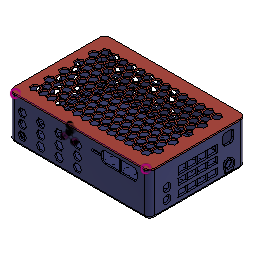
M5xxx (Autodesk Fusion 360 design; units mm, degrees)
Autodesk Fusion 360 part; units mm, degrees
note: some values were not read from the file. Set by a fixed rule: which face or edge a step refers to.
(part 1 of 4)
sketch "Sketch2" plane through (0, 0, 0) normal (0, 0, 1) x (1, 0, 0) in component "PCB-M5000"
  line L0 (110, -75) -> (-110, -75)
  line L1 (-110, -75) -> (-110, 75)
  line L2 (-110, 75) -> (110, 75)
  line L3 (110, 75) -> (110, -75)
  line L4 (110, -75) -> (-110, 75) construction
  line L5 (-110, -75) -> (110, 75) construction
  circle A0 centre (-105, 70) radius 1.75
  circle A1 centre (105, 70) radius 1.75
  circle A2 centre (105, -70) radius 1.75
  circle A3 centre (15, -70) radius 1.75
  circle A4 centre (-105, -70) radius 1.75
  line L6 (0, 0) -> (0, 75) construction
  line L7 (0, 0) -> (-110, 0) construction
  line L8 (125, 32) -> (100, 32)
  line L9 (100, 32) -> (100, -32)
  line L10 (100, -32) -> (125, -32)
  line L11 (125, -32) -> (125, 32)
  line L12 (125, 32) -> (100, -32) construction
  line L13 (100, 32) -> (125, -32) construction
  line L14 (110, -56) -> (97, -56)
  line L15 (97, -56) -> (97, -44)
  line L16 (97, -44) -> (110, -44)
  line L17 (110, -44) -> (110, -56)
  line L18 (110, -56) -> (97, -44) construction
  line L19 (97, -56) -> (110, -44) construction
  line L20 (-110, -62.5) -> (-103, -62.5)
  line L21 (-103, -62.5) -> (-103, -57.5)
  line L22 (-103, -57.5) -> (-110, -57.5)
  line L23 (-110, -57.5) -> (-110, -62.5)
  line L24 (-110, -62.5) -> (-103, -57.5) construction
  line L25 (-103, -62.5) -> (-110, -57.5) construction
  point P0 (112.5, 0)
  point P1 (103.5, -50)
  point P2 (-106.5, -60)
  dimension "d1" = 220
  dimension "d2" = 150
  dimension "d3" = 5
  dimension "d4" = 5
  dimension "d5" = 3.5
  dimension "d6" = 90
  dimension "d10" = 64
  dimension "d11" = 25
  dimension "d13" = 10
  dimension "d18" = 12
  dimension "d19" = 13
  dimension "d20" = 25
  dimension "d26" = 7
  dimension "d27" = 15
  dimension "d28" = 5
  constraint perpendicular L0 L1
  constraint parallel L0 L2
  constraint parallel L1 L3
  constraint horizontal L0
  constraint coincident L4 L6.start
  constraint coincident L5 L6.start
  constraint coincident L6.start L7.start
  constraint equal A3 A4
  constraint equal A2 A3
  constraint equal A1 A2
  constraint equal A0 A1
  constraint midpoint L2 L6.end
  constraint midpoint L1 L7.end
  constraint symmetric A0.centre A1.centre L6
  constraint symmetric A0.centre A4.centre L7
  constraint symmetric A2.centre A4.centre L6
  constraint horizontal A2.centre A3.centre
  constraint perpendicular L8 L9
  constraint parallel L8 L10
  constraint parallel L9 L11
  constraint horizontal L8
  constraint coincident L12 P0
  constraint coincident L13 P0
  constraint horizontal L6.start P0
  constraint perpendicular L14 L15
  constraint parallel L14 L16
  constraint parallel L15 L17
  constraint horizontal L14
  constraint coincident L3 L14.start
  constraint coincident L18 P1
  constraint coincident L19 P1
  constraint perpendicular L20 L21
  constraint parallel L20 L22
  constraint parallel L21 L23
  constraint horizontal L20
  constraint coincident L1 L20.start
  constraint coincident L24 P2
  constraint coincident L25 P2
  measures "d1" distance of L1.end L2.end
  measures "d2" distance of L0.end L1.end
  measures "d3" distance of L1 A0.centre
  measures "d4" distance of L2 A0.centre
  measures "d5" diameter of A0
  measures "d6" distance of A2.centre A3.centre
  measures "d10" distance of L8.end L9.end
  measures "d11" distance of L9.end L10.end
  measures "d13" distance of L3 L9
  measures "d18" distance of L14.end L15.end
  measures "d19" distance of L14.start L14.end
  measures "d20" distance of L0 P1
  measures "d26" distance of L21.end L22.end
  measures "d27" distance of L0 P2
  measures "d28" distance of L20.end L21.end
extrude "Extrude1" add sketch "Sketch2" against normal blind 1.6 contours L0 L1 L2 L3 L8 L9 L10 L14 L15 L16 L20 L21 L22 | L3 L14 L15 L16 L17 | L1 L20 L21 L22 L23 | L3 L8 L9 L10 makes body 1 in component "PCB-M5000"
extrude "Extrude2" add sketch "Sketch2" along normal blind 10.4 contours L3 L8 L9 L10 | L3 L8 L10 L11 bodies 1 in component "PCB-M5000"
fillet "Fillet1" radius 5 4 edges at (110, -75, -0.8) (-110, -75, -0.8) (-110, 75, -0.8) (110, 75, -0.8) on bodies 1 in component "PCB-M5000"
extrude "Extrude4" add sketch "Sketch2" along normal blind 11 contours L3 L14 L15 L16 L17 bodies 1 in component "PCB-M5000"
sketch "Sketch3" plane through (110, 0, 0) normal (1, 0, 0) x (0, 1, 0) in component "PCB-M5000"
  line L0 (-32, 0) -> (-44, 0)
  line L1 (-44, 0) -> (-44, 11)
  line L2 (-44, 11) -> (-56, 11)
  line L3 (-56, 11) -> (-56, 0)
  line L4 (-56, 0) -> (-70, 0)
  line L5 (-70, 0) -> (-70, -1.6)
  line L6 (-70, -1.6) -> (70, -1.6)
  circle A0 centre (-50, 6.5) radius 4.5
  line L7 (-50, 6.5) -> (-50, 11) construction
  line L8 (70, -1.6) -> (70, 0)
  line L9 (70, 0) -> (32, 0)
  line L10 (32, 0) -> (-32, 0)
  dimension "d23" = 9
  constraint tangent L2 A0
  constraint coincident A0.centre L7.start
  constraint midpoint L2 L7.end
  constraint vertical L7
  measures "d23" diameter of A0
extrude "Extrude5" add sketch "Sketch3" along normal blind 10 contours A0 bodies 1 in component "PCB-M5000"
extrude "Extrude6" add sketch "Sketch2" along normal blind 7.5 contours L1 L20 L21 L22 L23 bodies 1 in component "PCB-M5000"
sketch "Sketch4" plane through (-110, 0, 0) normal (-1, 0, 0) x (0, -1, 0) in component "PCB-M5000"
  line L0 (-70, 0) -> (-70, -1.6)
  line L1 (-70, -1.6) -> (70, -1.6)
  line L2 (70, -1.6) -> (70, 0)
  line L3 (70, 0) -> (62.5, 0)
  line L4 (62.5, 0) -> (62.5, 7.5)
  line L5 (62.5, 7.5) -> (57.5, 7.5)
  line L6 (57.5, 7.5) -> (57.5, 0)
  line L7 (57.5, 0) -> (-70, 0)
  circle A0 centre (60, 7.5) radius 1.75
  point P0 (60, 0)
  dimension "d31" = 3.5
  dimension "d243" = 7.5
  constraint vertical A0.centre P0
  measures "d31" diameter of A0
  measures "d243" distance of A0.centre P0
extrude "Extrude7" add sketch "Sketch4" along normal blind 10 contours L5 A0 | L5 A0 bodies 1 in component "PCB-M5000"
ref_plane "WorkPlane1" through (0, 0, 31.6) normal (0, 0, 1) x (1, 0, 0) in component "M2000"
sketch "Sketch1" plane through (0, 0, 31.6) normal (0, 0, 1) x (1, 0, 0) in component "M2000"
  line L0 (110, -75) -> (10, -75)
  line L1 (10, -75) -> (10, 75)
  line L2 (10, 75) -> (110, 75)
  line L3 (110, 75) -> (110, -75)
  line L4 (110, -75) -> (10, 75) construction
  line L5 (10, -75) -> (110, 75) construction
  line L6 (-105, 75) -> (105, 75)
  line L7 (105, -75) -> (-105, -75)
  line L8 (110, 70) -> (110, 32)
  circle A0 centre (105, -70) radius 1.75
  circle A1 centre (15, -70) radius 1.75
  circle A2 centre (105, 70) radius 1.75
  line L9 (125, -32) -> (125, 32)
  line L10 (125, 32) -> (100, 32)
  line L11 (100, 32) -> (100, -32)
  line L12 (100, -32) -> (125, -32)
  line L13 (95, -75) -> (35, -75)
  line L14 (35, -75) -> (35, -55)
  line L15 (35, -55) -> (95, -55)
  line L16 (95, -55) -> (95, -75)
  line L17 (95, -75) -> (35, -55) construction
  line L18 (35, -75) -> (95, -55) construction
  line L19 (110, 40) -> (90, 40)
  line L20 (90, 40) -> (90, 60)
  line L21 (90, 60) -> (110, 60)
  line L22 (110, 60) -> (110, 40)
  line L23 (110, 40) -> (90, 60) construction
  line L24 (90, 40) -> (110, 60) construction
  line L25 (34.5, -75) -> (19.5, -75)
  line L26 (19.5, -75) -> (19.5, -70)
  line L27 (19.5, -70) -> (34.5, -70)
  line L28 (34.5, -70) -> (34.5, -75)
  line L29 (34.5, -75) -> (19.5, -70) construction
  line L30 (19.5, -75) -> (34.5, -70) construction
  circle A3 centre (15, -60) radius 1.6
  point P0 (60, 0)
  point P1 (65, -65)
  point P2 (100, 50)
  point P3 (27, -72.5)
  dimension "d35" = 100
  dimension "d40" = 60
  dimension "d52" = 20
  dimension "d53" = 20
  dimension "d54" = 25
  dimension "d60" = 5
  dimension "d62" = 3.2
  dimension "d63" = 5
  dimension "d64" = 15
  dimension "d67" = 55
  dimension "d68" = 20
  dimension "d69" = 15
  dimension "d70" = 17
  constraint perpendicular L0 L1
  constraint parallel L0 L2
  constraint parallel L1 L3
  constraint horizontal L0
  constraint coincident L4 P0
  constraint coincident L5 P0
  constraint collinear L2 L6
  constraint collinear L0 L7
  constraint collinear L3 L8
  constraint perpendicular L13 L14
  constraint parallel L13 L15
  constraint parallel L14 L16
  constraint horizontal L13
  constraint coincident L17 P1
  constraint coincident L18 P1
  constraint midpoint L17 P1
  constraint coincident L0 L13.start
  constraint perpendicular L19 L20
  constraint parallel L19 L21
  constraint parallel L20 L22
  constraint horizontal L19
  constraint coincident L8 L19.start
  constraint coincident L23 P2
  constraint coincident L24 P2
  constraint perpendicular L25 L26
  constraint parallel L25 L27
  constraint parallel L26 L28
  constraint horizontal L25
  constraint coincident L29 P3
  constraint coincident L30 P3
  constraint coincident L27.end L28.start
  constraint coincident L7 L13.end
  constraint coincident L13.end L14.start
  constraint coincident L0 L25.end
  measures "d35" distance of L1.end L2.end
  measures "d40" distance of L14.end L15.end
  measures "d52" distance of L19.end L20.end
  measures "d53" distance of L19.start L19.end
  measures "d54" distance of L2 P2
  measures "d60" distance of L25.end L26.end
  measures "d62" diameter of A3
  measures "d63" distance of L1 A3.centre
  measures "d64" distance of L0 A3.centre
  measures "d67" distance of L1 P1
  measures "d68" distance of L14.end L13.end
  measures "d69" distance of L25.start L25.end
  measures "d70" horizontal distance of L0.end P3
extrude "Extrude1'" add sketch "Sketch1" along normal blind 1.6 separate body contours L0 L1 L2 L3 L6 L7 L8 L10 L11 L12 L14 L15 L16 L19 L20 L21 L26 L27 L28 | L3 L10 L11 L12 | L0 L7 L13 L14 L15 L16 | L3 L8 L19 L20 L21 L22 | L0 L7 L25 L26 L27 L28 | A3 makes body 2 in component "M2000"
extrude "Extrude2'" add sketch "Sketch1" along normal blind 12 contours L3 L10 L11 L12 | L3 L9 L10 L12 bodies 2 in component "M2000"
extrude "Extrude3" add sketch "Sketch1" along normal blind 20 from surface at 1.6 contours L0 L7 L13 L14 L15 L16 | L3 L8 L19 L20 L21 L22 bodies 2 in component "M2000"
extrude "Extrude6'" add sketch "Sketch1" along normal blind 35 contours A3 bodies 2 in component "M2000"
sketch "Sketch2 (2)" plane through (0, -75, 0) normal (0, -1, 0) x (1, 0, 0) in component "M2000"
  line L0 (10, 31.6) -> (110, 31.6)
  line L1 (110, 33.2) -> (95, 33.2)
  line L2 (95, 33.2) -> (95, 53.2)
  line L3 (95, 53.2) -> (35, 53.2)
  line L4 (35, 53.2) -> (35, 33.2)
  line L5 (35, 33.2) -> (10, 33.2)
  line L6 (10, 33.2) -> (10, 31.6)
  line L7 (93.8, 53.2) -> (36.2, 53.2)
  line L8 (36.2, 53.2) -> (36.2, 34.2)
  line L9 (36.2, 34.2) -> (93.8, 34.2)
  line L10 (93.8, 34.2) -> (93.8, 53.2)
  line L11 (93.8, 53.2) -> (36.2, 34.2) construction
  line L12 (36.2, 53.2) -> (93.8, 34.2) construction
  line L13 (110, 31.6) -> (110, 33.2)
  point P0 (65, 43.7)
  dimension "d46" = 1.2
  dimension "d47" = 1.2
  dimension "d48" = 19
  constraint perpendicular L7 L8
  constraint parallel L7 L9
  constraint parallel L8 L10
  constraint horizontal L7
  constraint coincident L3 L7.start
  constraint coincident L11 P0
  constraint coincident L12 P0
  measures "d46" distance of L2 L10
  measures "d47" distance of L4 L8
  measures "d48" distance of L7 L9
extrude "Extrude4'" add sketch "Sketch2 (2)" along normal blind 10 contours L3 L7 L8 L9 L10 bodies 2 in component "M2000"
sketch "Sketch3 (2)" plane through (110, 0, 0) normal (1, 0, 0) x (0, 1, 0) in component "M2000"
  line L0 (32, 31.6) -> (75, 31.6)
  line L1 (75, 31.6) -> (75, 33.2)
  line L2 (75, 33.2) -> (60, 33.2)
  line L3 (60, 33.2) -> (60, 53.2)
  line L4 (60, 53.2) -> (40, 53.2)
  line L5 (40, 53.2) -> (40, 33.2)
  line L6 (40, 33.2) -> (32, 33.2)
  line L7 (32, 33.2) -> (32, 31.6)
  line L8 (59, 53.2) -> (41, 53.2)
  line L9 (41, 53.2) -> (41, 34.2)
  line L10 (41, 34.2) -> (59, 34.2)
  line L11 (59, 34.2) -> (59, 53.2)
  line L12 (59, 53.2) -> (41, 34.2) construction
  line L13 (41, 53.2) -> (59, 34.2) construction
  point P0 (50, 43.7)
  dimension "d55" = 19
  dimension "d56" = 1
  dimension "d57" = 1
  constraint perpendicular L8 L9
  constraint parallel L8 L10
  constraint parallel L9 L11
  constraint horizontal L8
  constraint coincident L4 L8.start
  constraint coincident L12 P0
  constraint coincident L13 P0
  measures "d55" distance of L8.start L10.end
  measures "d56" distance of L3 L11
  measures "d57" distance of L5 L9
extrude "Extrude5'" add sketch "Sketch3 (2)" along normal blind 10 contours L4 L8 L9 L10 L11 bodies 2 in component "M2000"
fillet "Fillet1'" radius 5 8 edges at (36.2, -80, 53.2) (36.2, -80, 34.2) (93.8, -80, 34.2) (93.8, -80, 53.2) (115, 41, 53.2) (115, 59, 53.2) (115, 59, 34.2) (115, 41, 34.2) on bodies 2 in component "M2000"
fillet "Fillet2" radius 5 4 edges at (10, -75, 32.4) (10, 75, 32.4) (110, 75, 32.4) (110, -75, 32.4) on bodies 2 in component "M2000"
extrude "Extrude7'" add sketch "Sketch1" along normal blind 12.6 from surface at 1.6 contours L0 L7 L25 L26 L27 L28 bodies 2 in component "M2000"
sketch "Sketch4 (2)" plane through (0, -75, 0) normal (0, -1, 0) x (1, 0, 0) in component "M2000"
  line L0 (19.5, 33.2) -> (15, 33.2)
  line L1 (15, 33.2) -> (15, 31.6)
  line L2 (15, 31.6) -> (105, 31.6)
  line L3 (105, 33.2) -> (95, 33.2)
  line L4 (95, 33.2) -> (95, 53.2)
  line L5 (95, 53.2) -> (88.8, 53.2)
  arc A0 (93.8, 48.2) -> (88.8, 53.2) centre (88.8, 48.2) ccw
  line L6 (93.8, 48.2) -> (93.8, 39.2)
  arc A1 (88.8, 34.2) -> (93.8, 39.2) centre (88.8, 39.2) ccw
  line L7 (88.8, 34.2) -> (41.2, 34.2)
  arc A2 (36.2, 39.2) -> (41.2, 34.2) centre (41.2, 39.2) ccw
  line L8 (36.2, 39.2) -> (36.2, 48.2)
  arc A3 (41.2, 53.2) -> (36.2, 48.2) centre (41.2, 48.2) ccw
  line L9 (41.2, 53.2) -> (35, 53.2)
  line L10 (35, 53.2) -> (35, 33.2)
  line L11 (35, 33.2) -> (34.5, 33.2)
  line L12 (34.5, 33.2) -> (34.5, 45.8)
  line L13 (34.5, 45.8) -> (19.5, 45.8)
  line L14 (19.5, 45.8) -> (19.5, 33.2)
  line L15 (21.4, 42) -> (32.6, 42)
  arc A4 (32.6, 42) -> (32.6, 45.8) centre (32.6, 43.9) ccw
  line L16 (32.6, 45.8) -> (21.4, 45.8)
  arc A5 (21.4, 45.8) -> (21.4, 42) centre (21.4, 43.9) ccw
  line L17 (21.4, 43.9) -> (32.6, 43.9) construction
  line L18 (27, 43.9) -> (27, 31.6) construction
  line L19 (105, 31.6) -> (105, 33.2)
  point P0 (27, 31.6)
  dimension "d76" = 3.8
  constraint tangent L15 A4
  constraint tangent A4 L16
  constraint parallel L15 L16
  constraint tangent L16 A5
  constraint tangent L15 A5
  constraint parallel L0 L17
  constraint midpoint L17 L18.start
  constraint coincident P0 L18.end
  constraint vertical L18
  constraint coincident L13 L16.end
  constraint tangent L12 A4
  measures "d76" diameter of A4
extrude "Extrude8" add sketch "Sketch4 (2)" along normal blind 10 contours L13 L15 A4 L16 A5 bodies 2 in component "M2000"
ref_plane "WorkPlane1" through (0, 0, -7.6) normal (0, 0, -1) x (-1, 0, 0) in component "M5xxx-base"
sketch "Sketch1 (2)" plane through (7.5, 0, -7.6) normal (0, 0, -1) x (1, 0, 0) in component "M5xxx-base"
  line L0 (97.5, 75) -> (-112.5, 75)
  arc A0 (102.5, 70) -> (97.5, 75) centre (97.5, 70) ccw
  arc A1 (-112.5, 75) -> (-117.5, 70) centre (-112.5, 70) ccw
  arc A2 (-117.5, -70) -> (-112.5, -75) centre (-112.5, -70) ccw
  line L1 (-112.5, -75) -> (97.5, -75)
  circle A3 centre (-112.5, -70) radius 1.75 construction
  circle A4 centre (97.5, -70) radius 1.75 construction
  arc A5 (97.5, -75) -> (102.5, -70) centre (97.5, -70) ccw
  circle A6 centre (-112.5, 70) radius 1.75 construction
  circle A7 centre (7.5, 70) radius 1.75 construction
  circle A8 centre (97.5, 70) radius 1.75 construction
  line L2 (102.5, 70) -> (102.5, -70)
  line L3 (103.5, 70) -> (103.5, -70)
  arc A9 (97.5, -76) -> (103.5, -70) centre (97.5, -70) ccw
  line L4 (-112.5, -76) -> (97.5, -76)
  arc A10 (-118.5, -70) -> (-112.5, -76) centre (-112.5, -70) ccw
  line L5 (-118.5, 60) -> (-118.5, -70)
  line L6 (-118.5, 70) -> (-118.5, 60)
  arc A11 (-112.5, 76) -> (-118.5, 70) centre (-112.5, 70) ccw
  line L7 (97.5, 76) -> (-112.5, 76)
  arc A12 (103.5, 70) -> (97.5, 76) centre (97.5, 70) ccw
  arc A13 (97.5, -78.4) -> (105.9, -70) centre (97.5, -70) ccw
  line L8 (105.9, 70) -> (105.9, -70)
  arc A14 (105.9, 70) -> (97.5, 78.4) centre (97.5, 70) ccw
  line L9 (97.5, 78.4) -> (-112.5, 78.4)
  arc A15 (-112.5, 78.4) -> (-120.9, 70) centre (-112.5, 70) ccw
  line L10 (-120.9, 70) -> (-120.9, 60)
  line L11 (-120.9, 60) -> (-120.9, -70)
  arc A16 (-120.9, -70) -> (-112.5, -78.4) centre (-112.5, -70) ccw
  line L12 (-112.5, -78.4) -> (97.5, -78.4)
  arc A17 (97.5, -72) -> (99.5, -70) centre (97.5, -70) ccw
  line L13 (99.5, 70) -> (99.5, -70)
  arc A18 (99.5, 70) -> (97.5, 72) centre (97.5, 70) ccw
  line L14 (97.5, 72) -> (-112.5, 72)
  arc A19 (-112.5, 72) -> (-114.5, 70) centre (-112.5, 70) ccw
  line L15 (-114.5, 70) -> (-114.5, 60)
  line L16 (-114.5, 60) -> (-114.5, -70)
  arc A20 (-114.5, -70) -> (-112.5, -72) centre (-112.5, -70) ccw
  line L17 (-112.5, -72) -> (97.5, -72)
  circle A21 centre (97.5, -70) radius 5
  circle A22 centre (97.5, 70) radius 5
  circle A23 centre (-112.5, 70) radius 5
  circle A24 centre (-112.5, -70) radius 5
  circle A25 centre (7.5, 70) radius 5
  line L18 (96.75, -68.701) -> (96, -70)
  line L19 (96, -70) -> (96.75, -71.299)
  line L20 (96.75, -71.299) -> (98.25, -71.299)
  line L21 (98.25, -71.299) -> (99, -70)
  line L22 (99, -70) -> (98.25, -68.701)
  line L23 (98.25, -68.701) -> (96.75, -68.701)
  line L24 (96, 70) -> (96.75, 68.701)
  line L25 (96.75, 68.701) -> (98.25, 68.701)
  line L26 (98.25, 68.701) -> (99, 70)
  line L27 (99, 70) -> (98.25, 71.299)
  line L28 (98.25, 71.299) -> (96.75, 71.299)
  line L29 (96.75, 71.299) -> (96, 70)
  line L30 (8.25, 71.299) -> (6.75, 71.299)
  line L31 (6.75, 71.299) -> (6, 70)
  line L32 (6, 70) -> (6.75, 68.701)
  line L33 (6.75, 68.701) -> (8.25, 68.701)
  line L34 (8.25, 68.701) -> (9, 70)
  line L35 (9, 70) -> (8.25, 71.299)
  line L36 (-111.75, 71.299) -> (-113.25, 71.299)
  line L37 (-113.25, 71.299) -> (-114, 70)
  line L38 (-114, 70) -> (-113.25, 68.701)
  line L39 (-113.25, 68.701) -> (-111.75, 68.701)
  line L40 (-111.75, 68.701) -> (-111, 70)
  line L41 (-111, 70) -> (-111.75, 71.299)
  line L42 (-111.75, -68.701) -> (-113.25, -68.701)
  line L43 (-113.25, -68.701) -> (-114, -70)
  line L44 (-114, -70) -> (-113.25, -71.299)
  line L45 (-113.25, -71.299) -> (-111.75, -71.299)
  line L46 (-111.75, -71.299) -> (-111, -70)
  line L47 (-111, -70) -> (-111.75, -68.701)
  line L48 (-112.5, -78.4) -> (-114.5, -78.4)
  arc A26 (-122.8999, -69.9653) -> (-114.5, -78.4) centre (-114.5, -70) ccw
  arc A27 (-120.5, -70) -> (-114.5, -76) centre (-114.5, -70) ccw
  line L49 (-114.5, -76) -> (-112.5, -76)
  line L50 (0, 0) -> (-114.5, 0) construction
  line L51 (-122.8999, -69.9653) -> (-122.8999, 0)
  line L52 (-120.5, -70) -> (-120.5, 0)
  line L53 (-112.5, 78.4) -> (-114.5, 78.4)
  line L54 (-114.5, 76) -> (-112.5, 76)
  arc A28 (-114.5, 76) -> (-120.5, 70) centre (-114.5, 70) ccw
  arc A29 (-114.5, 78.4) -> (-122.8999, 69.9653) centre (-114.5, 70) ccw
  line L55 (-120.5, 70) -> (-120.5, 0)
  line L56 (-122.8999, 69.9653) -> (-122.8999, 0)
  arc A30 (106.9, 70) -> (98.5, 78.4) centre (98.5, 70) ccw
  line L57 (98.5, 78.4) -> (97.5, 78.4)
  line L58 (106.9, 70) -> (106.9, 0)
  line L59 (106.9, -70) -> (106.9, 0)
  arc A31 (98.5, -78.4) -> (106.9, -70) centre (98.5, -70) ccw
  line L60 (98.5, -78.4) -> (97.5, -78.4)
  point P0 (97.5, -70)
  point P1 (97.5, 70)
  point P2 (7.5, 70)
  point P3 (-112.5, 70)
  point P4 (-112.5, -70)
  dimension "d85" = 10
  dimension "d86" = 1.5
  dimension "d87" = 1.5
  dimension "d88" = 1.5
  dimension "d89" = 1.5
  dimension "d90" = 1.5
  dimension "d181" = 2
  dimension "d182" = 8.4
  dimension "d196" = 8.4
  dimension "d197" = 1
  constraint coincident A0.start L2.start
  constraint coincident A5.end L2.end
  constraint concentric A4 A21
  constraint concentric A0 A22
  constraint concentric A1 A23
  constraint concentric A2 A24
  constraint concentric A7 A25
  constraint equal A23 A25
  constraint equal A23 A24
  constraint equal A21 A24
  constraint equal A21 A22
  constraint coincident P0 A4.centre
  constraint coincident P1 A0.centre
  constraint coincident P2 A7.centre
  constraint coincident P3 A1.centre
  constraint coincident P4 A2.centre
  constraint horizontal L42
  constraint horizontal L39
  constraint horizontal L33
  constraint horizontal L25
  constraint horizontal L23
  constraint parallel L12 L48
  constraint tangent A10 L49
  constraint coincident L48.end A26.end
  constraint coincident L50.start origin
  constraint coincident L16 L50.end
  constraint perpendicular L16 L50
  constraint tangent A27 L52
  constraint parallel L11 L52
  constraint parallel L51 L52
  constraint horizontal L50.end L52.end
  constraint horizontal L51.end L52.end
  constraint symmetric L4.start L50 A11.start
  constraint symmetric A16.end L50 L9.end
  constraint symmetric L48.end L50 L53.end
  constraint symmetric A26.start L50 A29.end
  constraint symmetric A26 L50 A29
  constraint symmetric A27.start L50 A28.end
  constraint symmetric A27.end L50 L54.start
  constraint symmetric A27 L50 A28
  constraint symmetric L50 L51.end L56.end
  constraint symmetric L50 L52.end L55.end
  constraint concentric A26 A27
  constraint tangent A27 L49
  constraint tangent L48 A26
  constraint tangent A14 L57
  constraint tangent A30 L57
  constraint parallel L8 L58
  constraint horizontal L50.start L58.end
  constraint symmetric A14.end L50 A13.start
  constraint symmetric L50 A30.start L59.start
  constraint symmetric L50 A30.end A31.start
  constraint symmetric L50 A30 A31
  constraint symmetric L50 L58.end L59.end
  constraint parallel L2 L3
  constraint concentric A5 A9
  constraint parallel L1 L4
  constraint concentric A2 A10
  constraint concentric A1 A11
  constraint parallel L0 L7
  constraint concentric A0 A12
  constraint tangent A11 L7
  constraint tangent L6 A11
  constraint tangent A10 L5
  constraint tangent L4 A10
  constraint tangent A9 L4
  constraint tangent L3 A9
  constraint tangent L7 A12
  constraint tangent L3 A12
  constraint concentric A5 A13
  constraint parallel L2 L8
  constraint concentric A0 A14
  constraint parallel L0 L9
  constraint concentric A1 A15
  constraint concentric A2 A16
  constraint parallel L1 L12
  constraint tangent L11 A16
  constraint tangent A15 L10
  constraint tangent A14 L9
  constraint tangent L8 A14
  constraint tangent A13 L8
  constraint tangent L9 A15
  constraint tangent A16 L12
  constraint tangent A13 L12
  constraint concentric A5 A17
  constraint parallel L2 L13
  constraint concentric A0 A18
  constraint parallel L0 L14
  constraint concentric A1 A19
  constraint concentric A2 A20
  constraint parallel L1 L17
  constraint tangent A20 L17
  constraint tangent A19 L15
  constraint tangent A18 L14
  constraint tangent A17 L17
  constraint tangent L14 A19
  constraint tangent L13 A18
  constraint tangent L16 A20
  constraint tangent A17 L13
  measures "d85" diameter of A21
  measures "d86" distance of L18.start P0
  measures "d87" distance of L24.start P1
  measures "d88" distance of L30.start P2
  measures "d89" distance of L36.start P3
  measures "d90" distance of L42.start P4
  measures "d181" distance of A16.end L48.end
  measures "d182" radius of A26
  measures "d196" radius of A30
  measures "d197" distance of A14.end A30.end
extrude "Extrude1''" add sketch "Sketch1 (2)" along normal blind 2 separate body contours L0 L14 A22 A25 | A0 L13 A18 L14 A22 | L0 L14 A23 A25 | L14 A25 | L2 L13 A21 A22 | L13 L14 L15 L16 L17 A21 A22 A23 A24 A25 | L13 A18 L14 A22 | A1 L14 A19 L15 A23 | L14 A25 | A5 A17 L13 L17 A21 | L14 A19 L15 A23 | L1 L17 A21 A24 | A17 L13 L17 A21 | A2 L16 A20 L17 A24 | L16 A20 L17 A24 | L3 A9 L4 A10 L5 L6 A11 L7 A12 | A10 L5 L6 A11 A27 L49 L52 L54 A28 L55 | L18 L19 L20 L21 L22 L23 | L24 L25 L26 L27 L28 L29 | L30 L31 L32 L33 L34 L35 | L36 L37 L38 L39 L40 L41 | L42 L43 L44 L45 L46 L47 makes body 3 in component "M5xxx-base"
extrude "Extrude3'" add sketch "Sketch1 (2)" against normal up to surface (6 mm away) contours A0 L13 A18 L14 A22 | L14 A25 | L13 A18 L14 A22 | A1 L14 A19 L15 A23 | L14 A25 | A5 A17 L13 L17 A21 | L14 A19 L15 A23 | A17 L13 L17 A21 | A2 L16 A20 L17 A24 | L16 A20 L17 A24 bodies 3 in component "M5xxx-base"
extrude "Extrude4''" add sketch "Sketch1 (2)" against normal blind 4 contours L0 L14 A22 A25 | A0 L13 A18 L14 A22 | L0 L14 A23 A25 | L2 L13 A21 A22 | A5 A17 L13 L17 A21 | L1 L17 A21 A24 | L3 A9 L4 A10 L5 L6 A11 L7 A12 | A10 L5 L6 A11 A27 L49 L52 L54 A28 L55 bodies 3 in component "M5xxx-base"
sketch "Sketch2 (3)" plane through (0, 0, -7.6) normal (0, 0, 1) x (1, 0, 0) in component "M5xxx-base"
  line L0 (-107.5, -72) -> (107.5, -72)
  line L1 (107.5, 72) -> (-107.5, 72)
  line L2 (-109.5, 5) -> (-109.5, -5)
  line L3 (109.5, -5) -> (109.5, 5)
  line L4 (109.5, 70) -> (109.5, -70)
  line L5 (-107, 65.4174) -> (-107, -65.4174)
  arc A0 (-100.4174, -72) -> (-107, -65.4174) centre (-105, -70) ccw
  line L6 (-100.4174, -72) -> (10.4174, -72)
  arc A1 (19.5826, -72) -> (10.4174, -72) centre (15, -70) ccw
  line L7 (19.5826, -72) -> (100.4174, -72)
  arc A2 (107, -65.4174) -> (100.4174, -72) centre (105, -70) ccw
  line L8 (107, -65.4174) -> (107, 65.4174)
  arc A3 (100.4174, 72) -> (107, 65.4174) centre (105, 70) ccw
  line L9 (100.4174, 72) -> (-100.4174, 72)
  arc A4 (-107, 65.4174) -> (-100.4174, 72) centre (-105, 70) ccw
  line L10 (0, 0) -> (0, 72) construction
  line L11 (0, 0) -> (107, 0) construction
  line L12 (-100.4174, -72) -> (10.4174, -72)
  arc A5 (19.5826, -72) -> (10.4174, -72) centre (15, -70) ccw
  line L13 (19.5826, -72) -> (100.4174, -72)
  arc A6 (107, -65.4174) -> (100.4174, -72) centre (105, -70) ccw
  line L14 (107, -65.4174) -> (107, 65.4174)
  arc A7 (100.4174, 72) -> (107, 65.4174) centre (105, 70) ccw
  line L15 (100.4174, 72) -> (-100.4174, 72)
  arc A8 (-107, 65.4174) -> (-100.4174, 72) centre (-105, 70) ccw
  line L16 (-107, 65.4174) -> (-107, -65.4174)
  arc A9 (-100.4174, -72) -> (-107, -65.4174) centre (-105, -70) ccw
  line L17 (4.6188, -8) -> (9.2376, 0)
  line L18 (9.2376, 0) -> (4.6188, 8)
  line L19 (4.6188, 8) -> (-4.6188, 8)
  line L20 (-4.6188, 8) -> (-9.2376, 0)
  line L21 (-9.2376, 0) -> (-4.6188, -8)
  line L22 (-4.6188, -8) -> (4.6188, -8)
  line L23 (-85.3812, -58) -> (-80.7624, -50)
  line L24 (-99.2376, -50) -> (-94.6188, -58)
  line L25 (-80.7624, -50) -> (-85.3812, -42)
  line L26 (-94.6188, -58) -> (-85.3812, -58)
  line L27 (-85.3812, -42) -> (-94.6188, -42)
  line L28 (-94.6188, -42) -> (-99.2376, -50)
  line L29 (-55.3812, -58) -> (-50.7624, -50)
  line L30 (-69.2376, -50) -> (-64.6188, -58)
  line L31 (-50.7624, -50) -> (-55.3812, -42)
  line L32 (-64.6188, -58) -> (-55.3812, -58)
  line L33 (-55.3812, -42) -> (-64.6188, -42)
  line L34 (-64.6188, -42) -> (-69.2376, -50)
  line L35 (-25.3812, -58) -> (-20.7624, -50)
  line L36 (-39.2376, -50) -> (-34.6188, -58)
  line L37 (-20.7624, -50) -> (-25.3812, -42)
  line L38 (-34.6188, -58) -> (-25.3812, -58)
  line L39 (-25.3812, -42) -> (-34.6188, -42)
  line L40 (-34.6188, -42) -> (-39.2376, -50)
  line L41 (4.6188, -58) -> (9.2376, -50)
  line L42 (-9.2376, -50) -> (-4.6188, -58)
  line L43 (9.2376, -50) -> (4.6188, -42)
  line L44 (-4.6188, -58) -> (4.6188, -58)
  line L45 (4.6188, -42) -> (-4.6188, -42)
  line L46 (-4.6188, -42) -> (-9.2376, -50)
  line L47 (34.6188, -58) -> (39.2376, -50)
  line L48 (20.7624, -50) -> (25.3812, -58)
  line L49 (39.2376, -50) -> (34.6188, -42)
  line L50 (25.3812, -58) -> (34.6188, -58)
  line L51 (34.6188, -42) -> (25.3812, -42)
  line L52 (25.3812, -42) -> (20.7624, -50)
  line L53 (64.6188, -58) -> (69.2376, -50)
  line L54 (50.7624, -50) -> (55.3812, -58)
  line L55 (69.2376, -50) -> (64.6188, -42)
  line L56 (55.3812, -58) -> (64.6188, -58)
  line L57 (64.6188, -42) -> (55.3812, -42)
  line L58 (55.3812, -42) -> (50.7624, -50)
  line L59 (94.6188, -58) -> (99.2376, -50)
  line L60 (80.7624, -50) -> (85.3812, -58)
  line L61 (99.2376, -50) -> (94.6188, -42)
  line L62 (85.3812, -58) -> (94.6188, -58)
  line L63 (94.6188, -42) -> (85.3812, -42)
  line L64 (85.3812, -42) -> (80.7624, -50)
  line L65 (-85.3812, -33) -> (-80.7624, -25)
  line L66 (-99.2376, -25) -> (-94.6188, -33)
  line L67 (-80.7624, -25) -> (-85.3812, -17)
  line L68 (-94.6188, -33) -> (-85.3812, -33)
  line L69 (-85.3812, -17) -> (-94.6188, -17)
  line L70 (-94.6188, -17) -> (-99.2376, -25)
  line L71 (-55.3812, -33) -> (-50.7624, -25)
  line L72 (-69.2376, -25) -> (-64.6188, -33)
  line L73 (-50.7624, -25) -> (-55.3812, -17)
  line L74 (-64.6188, -33) -> (-55.3812, -33)
  line L75 (-55.3812, -17) -> (-64.6188, -17)
  line L76 (-64.6188, -17) -> (-69.2376, -25)
  line L77 (-25.3812, -33) -> (-20.7624, -25)
  line L78 (-39.2376, -25) -> (-34.6188, -33)
  line L79 (-20.7624, -25) -> (-25.3812, -17)
  line L80 (-34.6188, -33) -> (-25.3812, -33)
  line L81 (-25.3812, -17) -> (-34.6188, -17)
  line L82 (-34.6188, -17) -> (-39.2376, -25)
  line L83 (4.6188, -33) -> (9.2376, -25)
  line L84 (-9.2376, -25) -> (-4.6188, -33)
  line L85 (9.2376, -25) -> (4.6188, -17)
  line L86 (-4.6188, -33) -> (4.6188, -33)
  line L87 (4.6188, -17) -> (-4.6188, -17)
  line L88 (-4.6188, -17) -> (-9.2376, -25)
  line L89 (34.6188, -33) -> (39.2376, -25)
  line L90 (20.7624, -25) -> (25.3812, -33)
  line L91 (39.2376, -25) -> (34.6188, -17)
  line L92 (25.3812, -33) -> (34.6188, -33)
  line L93 (34.6188, -17) -> (25.3812, -17)
  line L94 (25.3812, -17) -> (20.7624, -25)
  line L95 (64.6188, -33) -> (69.2376, -25)
  line L96 (50.7624, -25) -> (55.3812, -33)
  line L97 (69.2376, -25) -> (64.6188, -17)
  line L98 (55.3812, -33) -> (64.6188, -33)
  line L99 (64.6188, -17) -> (55.3812, -17)
  line L100 (55.3812, -17) -> (50.7624, -25)
  line L101 (94.6188, -33) -> (99.2376, -25)
  line L102 (80.7624, -25) -> (85.3812, -33)
  line L103 (99.2376, -25) -> (94.6188, -17)
  line L104 (85.3812, -33) -> (94.6188, -33)
  line L105 (94.6188, -17) -> (85.3812, -17)
  line L106 (85.3812, -17) -> (80.7624, -25)
  line L107 (-85.3812, -8) -> (-80.7624, 0)
  line L108 (-99.2376, 0) -> (-94.6188, -8)
  line L109 (-80.7624, 0) -> (-85.3812, 8)
  line L110 (-94.6188, -8) -> (-85.3812, -8)
  line L111 (-85.3812, 8) -> (-94.6188, 8)
  line L112 (-94.6188, 8) -> (-99.2376, 0)
  line L113 (-55.3812, -8) -> (-50.7624, 0)
  line L114 (-69.2376, 0) -> (-64.6188, -8)
  line L115 (-50.7624, 0) -> (-55.3812, 8)
  line L116 (-64.6188, -8) -> (-55.3812, -8)
  line L117 (-55.3812, 8) -> (-64.6188, 8)
  line L118 (-64.6188, 8) -> (-69.2376, 0)
  line L119 (-25.3812, -8) -> (-20.7624, 0)
  line L120 (-39.2376, 0) -> (-34.6188, -8)
  line L121 (-20.7624, 0) -> (-25.3812, 8)
  line L122 (-34.6188, -8) -> (-25.3812, -8)
  line L123 (-25.3812, 8) -> (-34.6188, 8)
  line L124 (-34.6188, 8) -> (-39.2376, 0)
  line L125 (34.6188, -8) -> (39.2376, 0)
  line L126 (20.7624, 0) -> (25.3812, -8)
  line L127 (39.2376, 0) -> (34.6188, 8)
  line L128 (25.3812, -8) -> (34.6188, -8)
  line L129 (34.6188, 8) -> (25.3812, 8)
  line L130 (25.3812, 8) -> (20.7624, 0)
  line L131 (64.6188, -8) -> (69.2376, 0)
  line L132 (50.7624, 0) -> (55.3812, -8)
  line L133 (69.2376, 0) -> (64.6188, 8)
  line L134 (55.3812, -8) -> (64.6188, -8)
  line L135 (64.6188, 8) -> (55.3812, 8)
  line L136 (55.3812, 8) -> (50.7624, 0)
  line L137 (94.6188, -8) -> (99.2376, 0)
  line L138 (80.7624, 0) -> (85.3812, -8)
  line L139 (99.2376, 0) -> (94.6188, 8)
  line L140 (85.3812, -8) -> (94.6188, -8)
  line L141 (94.6188, 8) -> (85.3812, 8)
  line L142 (85.3812, 8) -> (80.7624, 0)
  line L143 (-85.3812, 17) -> (-80.7624, 25)
  line L144 (-99.2376, 25) -> (-94.6188, 17)
  line L145 (-80.7624, 25) -> (-85.3812, 33)
  line L146 (-94.6188, 17) -> (-85.3812, 17)
  line L147 (-85.3812, 33) -> (-94.6188, 33)
  line L148 (-94.6188, 33) -> (-99.2376, 25)
  line L149 (-55.3812, 17) -> (-50.7624, 25)
  line L150 (-69.2376, 25) -> (-64.6188, 17)
  line L151 (-50.7624, 25) -> (-55.3812, 33)
  line L152 (-64.6188, 17) -> (-55.3812, 17)
  line L153 (-55.3812, 33) -> (-64.6188, 33)
  line L154 (-64.6188, 33) -> (-69.2376, 25)
  line L155 (-25.3812, 17) -> (-20.7624, 25)
  line L156 (-39.2376, 25) -> (-34.6188, 17)
  line L157 (-20.7624, 25) -> (-25.3812, 33)
  line L158 (-34.6188, 17) -> (-25.3812, 17)
  line L159 (-25.3812, 33) -> (-34.6188, 33)
  line L160 (-34.6188, 33) -> (-39.2376, 25)
  line L161 (4.6188, 17) -> (9.2376, 25)
  line L162 (-9.2376, 25) -> (-4.6188, 17)
  line L163 (9.2376, 25) -> (4.6188, 33)
  line L164 (-4.6188, 17) -> (4.6188, 17)
  line L165 (4.6188, 33) -> (-4.6188, 33)
  line L166 (-4.6188, 33) -> (-9.2376, 25)
  line L167 (34.6188, 17) -> (39.2376, 25)
  line L168 (20.7624, 25) -> (25.3812, 17)
  line L169 (39.2376, 25) -> (34.6188, 33)
  line L170 (25.3812, 17) -> (34.6188, 17)
  line L171 (34.6188, 33) -> (25.3812, 33)
  line L172 (25.3812, 33) -> (20.7624, 25)
  line L173 (64.6188, 17) -> (69.2376, 25)
  line L174 (50.7624, 25) -> (55.3812, 17)
  line L175 (69.2376, 25) -> (64.6188, 33)
  line L176 (55.3812, 17) -> (64.6188, 17)
  line L177 (64.6188, 33) -> (55.3812, 33)
  line L178 (55.3812, 33) -> (50.7624, 25)
  line L179 (94.6188, 17) -> (99.2376, 25)
  line L180 (80.7624, 25) -> (85.3812, 17)
  line L181 (99.2376, 25) -> (94.6188, 33)
  line L182 (85.3812, 17) -> (94.6188, 17)
  line L183 (94.6188, 33) -> (85.3812, 33)
  line L184 (85.3812, 33) -> (80.7624, 25)
  line L185 (-85.3812, 42) -> (-80.7624, 50)
  line L186 (-99.2376, 50) -> (-94.6188, 42)
  line L187 (-80.7624, 50) -> (-85.3812, 58)
  line L188 (-94.6188, 42) -> (-85.3812, 42)
  line L189 (-85.3812, 58) -> (-94.6188, 58)
  line L190 (-94.6188, 58) -> (-99.2376, 50)
  line L191 (-55.3812, 42) -> (-50.7624, 50)
  line L192 (-69.2376, 50) -> (-64.6188, 42)
  line L193 (-50.7624, 50) -> (-55.3812, 58)
  line L194 (-64.6188, 42) -> (-55.3812, 42)
  line L195 (-55.3812, 58) -> (-64.6188, 58)
  line L196 (-64.6188, 58) -> (-69.2376, 50)
  line L197 (-25.3812, 42) -> (-20.7624, 50)
  line L198 (-39.2376, 50) -> (-34.6188, 42)
  line L199 (-20.7624, 50) -> (-25.3812, 58)
  line L200 (-34.6188, 42) -> (-25.3812, 42)
  line L201 (-25.3812, 58) -> (-34.6188, 58)
  line L202 (-34.6188, 58) -> (-39.2376, 50)
  line L203 (4.6188, 42) -> (9.2376, 50)
  line L204 (-9.2376, 50) -> (-4.6188, 42)
  line L205 (9.2376, 50) -> (4.6188, 58)
  line L206 (-4.6188, 42) -> (4.6188, 42)
  line L207 (4.6188, 58) -> (-4.6188, 58)
  line L208 (-4.6188, 58) -> (-9.2376, 50)
  line L209 (34.6188, 42) -> (39.2376, 50)
  line L210 (20.7624, 50) -> (25.3812, 42)
  line L211 (39.2376, 50) -> (34.6188, 58)
  line L212 (25.3812, 42) -> (34.6188, 42)
  line L213 (34.6188, 58) -> (25.3812, 58)
  line L214 (25.3812, 58) -> (20.7624, 50)
  line L215 (64.6188, 42) -> (69.2376, 50)
  line L216 (50.7624, 50) -> (55.3812, 42)
  line L217 (69.2376, 50) -> (64.6188, 58)
  line L218 (55.3812, 42) -> (64.6188, 42)
  line L219 (64.6188, 58) -> (55.3812, 58)
  line L220 (55.3812, 58) -> (50.7624, 50)
  line L221 (94.6188, 42) -> (99.2376, 50)
  line L222 (80.7624, 50) -> (85.3812, 42)
  line L223 (99.2376, 50) -> (94.6188, 58)
  line L224 (85.3812, 42) -> (94.6188, 42)
  line L225 (94.6188, 58) -> (85.3812, 58)
  line L226 (85.3812, 58) -> (80.7624, 50)
  point P0 (-90, -50)
  point P1 (-60, -50)
  point P2 (-30, -50)
  point P3 (0, -50)
  point P4 (30, -50)
  point P5 (60, -50)
  point P6 (90, -50)
  point P7 (-90, -25)
  point P8 (-60, -25)
  point P9 (-30, -25)
  point P10 (0, -25)
  point P11 (30, -25)
  point P12 (60, -25)
  point P13 (90, -25)
  point P14 (-90, 0)
  point P15 (-60, 0)
  point P16 (-30, 0)
  point P17 (30, 0)
  point P18 (60, 0)
  point P19 (90, 0)
  point P20 (-90, 25)
  point P21 (-60, 25)
  point P22 (-30, 25)
  point P23 (0, 25)
  point P24 (30, 25)
  point P25 (60, 25)
  point P26 (90, 25)
  point P27 (-90, 50)
  point P28 (-60, 50)
  point P29 (-30, 50)
  point P30 (0, 50)
  point P31 (30, 50)
  point P32 (60, 50)
  point P33 (90, 50)
  dimension "d296" = 8
  dimension "d299" = 30
  dimension "d300" = 25
  constraint parallel L2 L3
  constraint coincident L3.end L4
  constraint midpoint L1 L10.end
  constraint midpoint L8 L11.end
  constraint horizontal L22
  constraint coincident L10.start L11.start
  measures "d296" distance of L10.start L22
extrude "Extrude5''" cut sketch "Sketch2 (3)" along normal blind 1 from surface at -2 contours L17 L18 L19 L20 L21 L22 | L23 L24 L25 L26 L27 L28 | L29 L30 L31 L32 L33 L34 | L35 L36 L37 L38 L39 L40 | L41 L42 L43 L44 L45 L46 | L47 L48 L49 L50 L51 L52 | L53 L54 L55 L56 L57 L58 | L59 L60 L61 L62 L63 L64 | L65 L66 L67 L68 L69 L70 | L71 L72 L73 L74 L75 L76 | L77 L78 L79 L80 L81 L82 | L83 L84 L85 L86 L87 L88 | L89 L90 L91 L92 L93 L94 | L95 L96 L97 L98 L99 L100 | L101 L102 L103 L104 L105 L106 | L107 L108 L109 L110 L111 L112 | L113 L114 L115 L116 L117 L118 | L119 L120 L121 L122 L123 L124 | L125 L126 L127 L128 L129 L130 | L131 L132 L133 L134 L135 L136 | L137 L138 L139 L140 L141 L142 | L143 L144 L145 L146 L147 L148 | L149 L150 L151 L152 L153 L154 | L155 L156 L157 L158 L159 L160 | L161 L162 L163 L164 L165 L166 | L167 L168 L169 L170 L171 L172 | L173 L174 L175 L176 L177 L178 | L179 L180 L181 L182 L183 L184 | L185 L186 L187 L188 L189 L190 | L191 L192 L193 L194 L195 L196 | L197 L198 L199 L200 L201 L202 | L203 L204 L205 L206 L207 L208 | L209 L210 L211 L212 L213 L214 | L215 L216 L217 L218 L219 L220 | L221 L222 L223 L224 L225 L226 bodies 3 in component "M5xxx-base"
extrude "Extrude6''" add sketch "Sketch1 (2)" along normal blind -66 and the other way blind -2 contours A13 L8 A14 L9 A15 L10 L11 A16 L12 | A13 L8 A14 A30 L57 L58 L59 A31 L60 | A15 L10 L11 A16 L48 A26 L51 L53 A29 L56 bodies 3 in component "M5xxx-base"
chamfer "Chamfer5" distance 2 angle 60 8 edges at (-112.952, 75.9274, -9.6) (-0.5, 78.4, -9.6) (111.9397, 75.9397, -9.6) (114.4, 0, -9.6) (111.9397, -75.9397, -9.6) (-0.5, -78.4, -9.6) (-112.952, -75.9274, -9.6) (-115.3999, 0, -9.6) measured on face at (-1.8729, 71.6, -9.6) measured on face at (-1.8729, 71.6, -9.6) measured on face at (-1.8729, 71.6, -9.6) measured on face at (-1.8729, 71.6, -9.6) measured on face at (-1.8729, 71.6, -9.6) measured on face at (-1.8729, 71.6, -9.6) measured on face at (-1.8729, 71.6, -9.6) measured on face at (-1.8729, 71.6, -9.6) on bodies 3 in component "M5xxx-base"